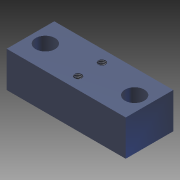
# Autodesk Inventor part: 13_0204_069
Saved by Autodesk Inventor 2012 SP1 (Build 160190100, 190)
## iProperties
Created: 2013-05-06
Part Number: 13_0204_069
Material: Default
Document SubType Name: Modeling
Designer: vogel
Density: 1 g/cm^3
Author: vogel
Autodesk Inventor part; units mm, degrees
ref_plane "YZ Plane" through (0, 0, 0) normal (1, 0, 0) x (0, 1, 0)
ref_plane "XZ Plane" through (0, 0, 0) normal (0, 1, 0) x (-1, 0, 0)
ref_plane "XY Plane" through (0, 0, 0) normal (0, 0, 1) x (1, 0, 0)
sketch "Skizze1" plane through (0, 0, 0) normal (0, 0, 1) x (1, 0, 0)
  line L0 (0, 0) -> (40, 0)
  line L1 (40, 0) -> (40, 16)
  line L2 (40, 16) -> (0, 16)
  line L3 (0, 16) -> (0, 0)
  dimension "d0" = 16
  dimension "d1" = 40
  constraints: 8 end point, 2 parallel, 1 horizontal, 1 perpendicular
  measures "d0" distance of L2.end L0.start
  measures "d1" distance of L0.start L0.end
extrude "Extrusion1" add sketch "Skizze1" along normal blind 12
sketch "Skizze2" plane through (0, 0, 12) normal (0, 0, 1) x (1, 0, 0)
  line L0 (40, 0) -> (0, 0) projected
  line L1 (0, 16) -> (40, 16) projected
  line L2 (20, 16) -> (20, 0)
  point P0 (20, 12)
  point P1 (20, 4)
  dimension "d4" = 4
  dimension "d5" = 8
  constraints: 2 end point, 2 midpoint, 2 point on line
  measures "d4" distance from line of L1 point (20, 12)
  measures "d5" distance of point (20, 4) point (20, 12)
hole "Bohrung1" at (20, 12, 12) at (20, 4, 12) direction (0, 0, -1) diameter 2.459 end through all thread size "M3x0.5" class "6H" standard "ISO Metric profile"
sketch "Skizze3" plane through (0, 0, 12) normal (0, 0, 1) x (1, 0, 0)
  line L0 (0, 0) -> (0, 16) projected
  line L1 (40, 0) -> (0, 0) projected
  line L2 (40, 16) -> (40, 0) projected
  line L3 (0, 16) -> (40, 16) projected
  line L4 (0, 8) -> (40, 8)
  line L5 (20, 16) -> (20, 0)
  point P0 (5, 8)
  point P1 (35, 8)
  dimension "d13" = 30
  constraints: 4 end point, 4 midpoint, 2 point on line, 1 symmetric about line
  measures "d13" distance of point (35, 8) point (5, 8)
hole "Bohrung2" at (5, 8, 12) at (35, 8, 12) direction (0, 0, -1) diameter 3.4 end through all counterbore diameter 6.5 counterbore depth 5
